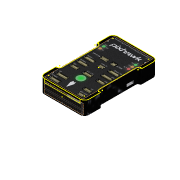
# Autodesk Inventor part: Pixhawk
Saved by Autodesk Inventor 2014 (Build 180170000, 170)
## iProperties
Created: 2014-12-16
Part Number: Pixhawk
Material: Generic
Document SubType Name: Modeling
Designer: Admin
Mass: 40000 g
Surface Area: 129.998 cm^2
Volume: 56.2293 cm^3
Density: 711.373 g/cm^3
Appearance: Default
Author: Admin
Autodesk Inventor part; units mm, degrees
ref_plane "YZ Plane" through (0, 0, 0) normal (1, 0, 0) x (0, 1, 0)
ref_plane "XZ Plane" through (0, 0, 0) normal (0, 1, 0) x (-1, 0, 0)
ref_plane "XY Plane" through (0, 0, 0) normal (0, 0, 1) x (1, 0, 0)
sketch "Sketch1" plane through (0, 0, 0) normal (0, 1, 0) x (-1, 0, 0)
  line L0 (-20, 41) -> (20, 41)
  line L1 (20, -41) -> (-20, -41)
  line L2 (-22, 20) -> (-22, -20)
  line L3 (22, 20) -> (22, -20)
  line L4 (24, -22) -> (23.5, -22)
  line L5 (-24, -22) -> (-23.5, -22)
  line L6 (-25, -36) -> (-25, -23.5)
  line L7 (-25, 23.5) -> (-25, 36)
  line L8 (23.5, 22) -> (24, 22)
  line L9 (-24, 22) -> (-23.5, 22)
  line L10 (25, 36) -> (25, 23.5)
  line L11 (25, -23.5) -> (25, -36)
  arc A0 (-20, 41) -> (-25, 36) centre (-20, 36) ccw
  arc A1 (25, 36) -> (20, 41) centre (20, 36) ccw
  arc A2 (-25, -36) -> (-20, -41) centre (-20, -36) ccw
  arc A3 (20, -41) -> (25, -36) centre (20, -36) ccw
  arc A4 (-22, 20) -> (-24, 22) centre (-24, 20) ccw
  arc A5 (-24, -22) -> (-22, -20) centre (-24, -20) ccw
  arc A6 (22, -20) -> (24, -22) centre (24, -20) ccw
  arc A7 (24, 22) -> (22, 20) centre (24, 20) ccw
  arc A8 (-25, 23.5) -> (-23.5, 22) centre (-23.5, 23.5) ccw
  arc A9 (23.5, 22) -> (25, 23.5) centre (23.5, 23.5) ccw
  arc A10 (25, -23.5) -> (23.5, -22) centre (23.5, -23.5) ccw
  arc A11 (-23.5, -22) -> (-25, -23.5) centre (-23.5, -23.5) ccw
  point P0 (0, 0)
  point P1 (25, -41)
  point P2 (25, 41)
  point P3 (-25, -41)
  dimension "d0" = 50
  dimension "d1" = 82
  dimension "d3" = 5
  dimension "d4" = 5
  dimension "d5" = 2
  dimension "d6" = 1.5
  constraints: 24 end point, 24 point on circle, 24 tangent, 12 centre point, 8 equal radius, 8 perpendicular, 6 equal length, 6 point on line, 1 horizontal
  measures "d0" distance of point (25, -41) point (-25, -41)
  measures "d1" distance of point (25, 41) point (25, -41)
  measures "d3" radius of A0
  measures "d4" radius of A2
  measures "d5" radius of A4
  measures "d6" radius of A8
extrude "Extrusion1" add sketch "Sketch1" along normal mid plane 15.5
chamfer "Chamfer1" distance 1 angle 45 6 edges at (22, 7.75, 0) (22.5858, 7.75, -21.4142) (22.5858, 7.75, 21.4142) (-22, 7.75, 0) (-22.5858, 7.75, 21.4142) (-22.5858, 7.75, -21.4142)
sketch "Sketch3" plane through (-20, 7.75, 41) normal (0, 0, 1) x (1, 0, 0)
  line L0 (0, -4.0516) -> (40, -4.0516)
  line L1 (40, -4.0516) -> (40, -14.4687)
  line L2 (40, -14.4687) -> (0, -14.4687)
  line L3 (0, -4.0516) -> (0, -14.4687)
  circle A0 centre (1.1708, -5.4188) radius 0.25
  circle A1 centre (1.1471, -9.2175) radius 0.25
  circle A2 centre (1.1471, -12.9073) radius 0.25
  circle A3 centre (4.4086, -5.4449) radius 0.25
  circle A4 centre (4.3852, -9.128) radius 0.25
  circle A5 centre (4.3848, -12.9334) radius 0.25
  circle A6 centre (7.7825, -5.4449) radius 0.25
  circle A7 centre (7.7587, -9.2436) radius 0.25
  circle A8 centre (7.7587, -12.9334) radius 0.25
  circle A9 centre (11.0203, -5.471) radius 0.25
  circle A10 centre (10.9965, -9.2697) radius 0.25
  circle A11 centre (10.9965, -12.9595) radius 0.25
  circle A12 centre (14.2234, -5.4823) radius 0.25
  circle A13 centre (14.1997, -9.281) radius 0.25
  circle A14 centre (14.1997, -12.9708) radius 0.25
  circle A15 centre (17.4612, -5.5084) radius 0.25
  circle A16 centre (17.4378, -9.1915) radius 0.25
  circle A17 centre (17.4374, -12.9969) radius 0.25
  circle A18 centre (20.8351, -5.5084) radius 0.25
  circle A19 centre (20.8113, -9.3071) radius 0.25
  circle A20 centre (20.8113, -12.9969) radius 0.25
  circle A21 centre (24.0729, -5.5345) radius 0.25
  circle A22 centre (24.0491, -9.3332) radius 0.25
  circle A23 centre (24.0491, -13.023) radius 0.25
  circle A24 centre (27.0517, -9.4065) radius 0.25
  circle A25 centre (27.0517, -13.0963) radius 0.25
  circle A26 centre (27.0755, -5.6078) radius 0.25
  circle A27 centre (30.2895, -13.1224) radius 0.25
  circle A28 centre (30.3132, -5.634) radius 0.25
  circle A29 centre (33.6634, -9.4326) radius 0.25
  circle A30 centre (33.6634, -13.1224) radius 0.25
  circle A31 centre (33.6872, -5.634) radius 0.25
  circle A32 centre (36.9012, -9.4587) radius 0.25
  circle A33 centre (36.9012, -13.1485) radius 0.25
  circle A34 centre (36.9249, -5.6601) radius 0.25
  circle A35 centre (30.2899, -9.3171) radius 0.25
  point P0 (0, 0)
  dimension "d13" = 0.5
  dimension "d14" = 0.5
  dimension "d15" = 0.5
  dimension "d16" = 0.5
  dimension "d17" = 0.5
  dimension "d18" = 0.5
  dimension "d19" = 0.5
  dimension "d20" = 0.5
  dimension "d21" = 0.5
  dimension "d22" = 0.5
  dimension "d23" = 0.5
  dimension "d24" = 0.5
  dimension "d31" = 0.5
  dimension "d32" = 0.5
  dimension "d33" = 0.5
  dimension "d34" = 0.5
  dimension "d35" = 0.5
  dimension "d36" = 0.5
  dimension "d37" = 0.5
  dimension "d38" = 0.5
  dimension "d39" = 0.5
  dimension "d40" = 0.5
  dimension "d41" = 0.5
  dimension "d42" = 0.5
  dimension "d43" = 0.5
  dimension "d44" = 0.5
  dimension "d45" = 0.5
  dimension "d46" = 0.5
  dimension "d47" = 0.5
  dimension "d48" = 0.5
  dimension "d49" = 0.5
  dimension "d50" = 0.5
  dimension "d51" = 0.5
  dimension "d52" = 0.5
  dimension "d53" = 0.5
  dimension "d54" = 0.5
  constraints: 36 centre point, 8 end point, 2 perpendicular
  measures "d13" diameter of A0
  measures "d14" diameter of A1
  measures "d15" diameter of A2
  measures "d16" diameter of A3
  measures "d17" diameter of A4
  measures "d18" diameter of A5
  measures "d19" diameter of A6
  measures "d20" diameter of A7
  measures "d21" diameter of A8
  measures "d22" diameter of A9
  measures "d23" diameter of A10
  measures "d24" diameter of A11
  measures "d31" diameter of A12
  measures "d32" diameter of A13
  measures "d33" diameter of A14
  measures "d34" diameter of A15
  measures "d35" diameter of A16
  measures "d36" diameter of A17
  measures "d37" diameter of A18
  measures "d38" diameter of A19
  measures "d39" diameter of A20
  measures "d40" diameter of A21
  measures "d41" diameter of A22
  measures "d42" diameter of A23
  measures "d43" diameter of A26
  measures "d44" diameter of A24
  measures "d45" diameter of A25
  measures "d46" diameter of A28
  measures "d47" diameter of A35
  measures "d48" diameter of A27
  measures "d49" diameter of A31
  measures "d50" diameter of A29
  measures "d51" diameter of A30
  measures "d52" diameter of A34
  measures "d53" diameter of A32
  measures "d54" diameter of A33
extrude "Extrusion2" cut sketch "Sketch3" against normal blind 6
sketch "Sketch4" plane through (20, 7.75, -41) normal (0, 0, -1) x (-1, 0, 0)
  line L0 (15.3879, -1.1055) -> (25.0213, -1.1055)
  line L1 (25.0213, -1.1055) -> (25.0213, -5.2702)
  line L2 (25.0213, -5.2702) -> (15.3879, -5.2702)
  line L3 (15.3879, -5.2702) -> (15.3879, -1.1055)
  point P0 (20, -7.75)
  constraints: 8 end point, 2 parallel, 1 horizontal, 1 perpendicular
extrude "Extrusion3" cut sketch "Sketch4" against normal blind 6
sketch "Sketch5" plane through (20, 7.75, -35) normal (0, 0, -1) x (-1, 0, 0)
  line L0 (15.3879, -1.1055) -> (25.0213, -1.1055) projected
  line L1 (15.3879, -5.2702) -> (15.3879, -1.1055) projected
  line L2 (25.0213, -5.2702) -> (15.3879, -5.2702) projected
  line L3 (25.0213, -1.1055) -> (25.0213, -5.2702) projected
  line L4 (15.3879, -3.9073) -> (25.0213, -3.9073)
  line L5 (25.0213, -3.9073) -> (25.0213, -4.6229)
  line L6 (25.0213, -4.6229) -> (15.3879, -4.6229)
  line L7 (15.3879, -4.6229) -> (15.3879, -3.9073)
  point P0 (20, -7.75)
  constraints: 8 end point, 2 parallel, 2 point on line, 1 horizontal, 1 perpendicular
extrude "Extrusion4" cut sketch "Sketch5" against normal blind 3 contours L0 L3 L4 L1 | L6 L3 L2 L1
sketch "Sketch6" plane through (22, -7.75, 20) normal (1, 0, 0) x (0, 0, -1)
  line L0 (29.2679, 5.7369) -> (37.2581, 5.7369)
  line L1 (37.2581, 5.7369) -> (37.2581, 2.6789)
  line L2 (37.2581, 2.6789) -> (29.2679, 2.6789)
  line L3 (29.2679, 2.6789) -> (29.2679, 5.7369)
  point P0 (20, 7.75)
  constraints: 8 end point, 2 parallel, 1 horizontal, 1 perpendicular
extrude "Extrusion5" cut sketch "Sketch6" against normal blind 3
sketch "Sketch7" plane through (0, 7.75, 0) normal (0, 1, 0) x (1, 0, 0)
  arc A0 (-24.8628, -22.8733) -> (-21, -20) centre (-24, -20) ccw projected
  arc A1 (-24.8628, -22.8733) -> (-25, -23.5) centre (-23.5, -23.5) ccw projected
  line L0 (-25, -23.5) -> (-25, -36) projected
  arc A2 (-25, -36) -> (-20, -41) centre (-20, -36) ccw projected
  line L1 (-20, -41) -> (20, -41) projected
  arc A3 (20, -41) -> (25, -36) centre (20, -36) ccw projected
  line L2 (25, -36) -> (25, -23.5) projected
  arc A4 (25, -23.5) -> (24.8628, -22.8733) centre (23.5, -23.5) ccw projected
  arc A5 (21, -20) -> (24.8628, -22.8733) centre (24, -20) ccw projected
  line L3 (21, 20) -> (21, -20) projected
  arc A6 (24.8628, 22.8733) -> (21, 20) centre (24, 20) ccw projected
  arc A7 (24.8628, 22.8733) -> (25, 23.5) centre (23.5, 23.5) ccw projected
  line L4 (25, 23.5) -> (25, 36) projected
  arc A8 (25, 36) -> (20, 41) centre (20, 36) ccw projected
  line L5 (20, 41) -> (-20, 41) projected
  arc A9 (-20, 41) -> (-25, 36) centre (-20, 36) ccw projected
  line L6 (-25, 36) -> (-25, 23.5) projected
  arc A10 (-25, 23.5) -> (-24.8628, 22.8733) centre (-23.5, 23.5) ccw projected
  arc A11 (-21, 20) -> (-24.8628, 22.8733) centre (-24, 20) ccw projected
  line L7 (-21, -20) -> (-21, 20) projected
  line L8 (-21.4799, 39.3573) -> (21.8643, 39.3573) construction
  line L9 (21.8643, 39.3573) -> (21.8643, -39.5227) construction
  line L10 (21.8643, -39.5227) -> (-21.4799, -39.5227) construction
  line L11 (-21.4799, -39.5227) -> (-21.4799, 39.3573) construction
  point P0 (0, 0)
  constraints: 2 other
sketch "Sketch8" plane through (-20, 7.75, 41) normal (0, 0, 1) x (1, 0, 0)
  line L0 (0, -4.0516) -> (40, -4.0516) projected
  line L1 (40, -4.0516) -> (40, 0) projected
  line L2 (0, 0) -> (40, 0) projected
  line L3 (0, 0) -> (0, -4.0516) projected
  line L4 (0, -2.4579) -> (43.4321, -2.4579) construction
  line L5 (43.4321, -2.4579) -> (43.4321, -14.2561) construction
  line L6 (43.4321, -14.2561) -> (0, -14.2561) construction
  line L7 (0, -14.2561) -> (0, -2.4579) construction
  point P0 (20, -7.75)
  constraints: 1 point on line, 2 other
body "Solid1"
